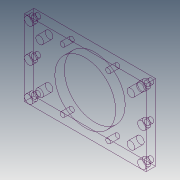
# Autodesk Inventor part: JF-AT-JC0014
Saved by Autodesk Inventor 2015 SP1 (Build 190203100, 203)
## iProperties
Created: 2010-04-29
Part Number: JF-AT-JC0014
Description: Clamper Plate
Document SubType Name: Modeling
Designer: S. Bassin
Density: 2.71 g/cm^3
Material: Aluminum-6061 (Anodized Black)
Mass: 89.7887 g
Surface Area: 133.388 cm^2
Volume: 33.1324 cm^3
Vendor: HHMI: JRC - ID&F
Appearance: Metal-AL-6061 (anodized black)
Revision Number: 0
Autodesk Inventor part; units mm, degrees
ref_plane "YZ Plane" through (0, 0, 0) normal (1, 0, 0) x (0, 1, 0)
ref_plane "XZ Plane" through (0, 0, 0) normal (0, 1, 0) x (-1, 0, 0)
ref_plane "XY Plane" through (0, 0, 0) normal (0, 0, 1) x (1, 0, 0)
sketch "Sketch1" plane through (0, 0, 0) normal (0, 0, 1) x (1, 0, 0)
  line L0 (-21.6696, 43.0812) -> (79.9304, 43.0812)
  line L1 (79.9304, 43.0812) -> (79.9304, -20.4188)
  line L2 (79.9304, -20.4188) -> (-21.6696, -20.4188)
  line L3 (-21.6696, -20.4188) -> (-21.6696, 43.0812)
  point P0 (0, 0)
  dimension "d0" = 101.6
  dimension "d1" = 63.5
  constraints: 8 end point
  measures "d0" distance between parallel lines of L1 L3
  measures "d1" distance between parallel lines of L2 L0
extrude "Extrusion1" add sketch "Sketch1" along normal blind 7.9375
sketch "Sketch3" plane through (0, 0, 7.9375) normal (0, 0, 1) x (1, 0, 0)
  line L0 (-21.6696, 43.0812) -> (79.9304, 43.0812) projected
  line L1 (-21.6696, -20.4188) -> (-21.6696, 43.0812) projected
  point P0 (0, 0)
  point P1 (29.1304, 11.3312)
  dimension "d15" = 31.75
  dimension "d16" = 50.8
  measures "d15" distance from line of L0 point (29.13, 11.331)
  measures "d16" distance from line of L1 point (29.13, 11.331)
hole "Hole2" at (29.1304, 11.3312, 7.9375) direction (0, 0, -1) diameter 50.8 end through all
sketch "Sketch4" plane through (0, 0, 7.9375) normal (0, 0, 1) x (1, 0, 0)
  line L0 (-21.6696, -20.4188) -> (-21.6696, 43.0812) projected
  line L1 (79.9304, -20.4188) -> (-21.6696, -20.4188) projected
  point P0 (0, 0)
  point P1 (10.0804, 36.7312)
  point P2 (10.0804, -14.0688)
  point P3 (48.1804, 36.7312)
  point P4 (48.1804, -14.0688)
  dimension "d24" = 50.8
  dimension "d25" = 6.35
  dimension "d26" = 38.1
  dimension "d27" = 31.75
  dimension "d28" = 31.75
  measures "d24" distance of point (10.08, 36.731) point (10.08, -14.069)
  measures "d25" distance from line of L1 point (10.08, -14.069)
  measures "d26" distance of point (48.18, 36.731) point (10.08, 36.731)
  measures "d27" distance from line of L0 point (10.08, 36.731)
  measures "d28" distance from line of L0 point (10.08, -14.069)
hole "Hole3" at (10.0804, 36.7312, 7.9375) at (10.0804, -14.0688, 7.9375) at (48.1804, 36.7312, 7.9375) at (48.1804, -14.0688, 7.9375) direction (0, 0, -1) diameter 3.9624 end through all thread size "10-32 UNF" class "2B" standard "ANSI Unified Screw Threads"
sketch "Sketch5" plane through (0, 0, 7.9375) normal (0, 0, 1) x (1, 0, 0)
  line L0 (79.9304, 43.0812) -> (79.9304, -20.4188) projected
  line L1 (-21.6696, 43.0812) -> (79.9304, 43.0812) projected
  line L2 (-21.6696, -20.4188) -> (-21.6696, 43.0812) projected
  line L3 (79.9304, -20.4188) -> (-21.6696, -20.4188) projected
  point P0 (0, 0)
  point P1 (-18.1136, 39.5252)
  point P2 (-18.1136, -16.8628)
  point P3 (76.3744, -16.8628)
  point P4 (76.3744, 39.5252)
  point P5 (-18.1136, 11.3312)
  point P6 (76.3744, 11.3312)
  dimension "d36" = 3.556
  dimension "d37" = 3.556
  dimension "d38" = 3.556
  dimension "d39" = 3.556
  dimension "d47" = 3.556
  dimension "d48" = 3.556
  dimension "d49" = 3.556
  dimension "d50" = 3.556
  dimension "d51" = 3.556
  dimension "d52" = 3.556
  dimension "d66" = 94.488
  dimension "d67" = 56.388
  measures "d36" distance from line of L2 point (-18.114, 39.525)
  measures "d37" distance from line of L1 point (-18.114, 39.525)
  measures "d38" distance from line of point (-18.114, -16.863) L3
  measures "d39" distance from line of L0 point (76.374, -16.863)
  measures "d47" distance from line of L2 point (-18.114, -16.863)
  measures "d48" distance from line of L2 point (-18.114, 11.331)
  measures "d49" distance from line of point (76.374, -16.863) L3
  measures "d50" distance from line of point (76.374, 11.331) L0
  measures "d51" distance from line of L0 point (76.374, 39.525)
  measures "d52" horizontal distance of L0.start point (76.374, 39.525)
  measures "d66" horizontal distance of point (76.374, -16.863) point (-18.114, 39.525)
  measures "d67" distance of point (-18.114, -16.863) point (-18.114, 39.525)
hole "Hole4" at (-18.1136, 39.5252, 7.9375) at (-18.1136, -16.8628, 7.9375) at (76.3744, -16.8628, 7.9375) at (76.3744, 39.5252, 7.9375) at (-18.1136, 11.3312, 7.9375) at (76.3744, 11.3312, 7.9375) direction (0, 0, -1) diameter 4.318 end through all counterbore diameter 6.985 counterbore depth 4.1656
sketch "Sketch6" plane through (0, 0, 7.9375) normal (0, 0, 1) x (1, 0, 0)
  line L0 (79.9304, 43.0812) -> (79.9304, -20.4188) projected
  line L1 (-21.6696, 43.0812) -> (79.9304, 43.0812) projected
  line L2 (-21.6696, -20.4188) -> (-21.6696, 43.0812) projected
  line L3 (79.9304, -20.4188) -> (-21.6696, -20.4188) projected
  point P0 (0, 0)
  point P1 (-8.9696, 30.3812)
  point P2 (-8.9696, -7.7188)
  point P3 (67.2304, 30.3812)
  point P4 (67.2304, -7.7188)
  dimension "d53" = 12.7
  dimension "d54" = 12.7
  dimension "d55" = 12.7
  dimension "d56" = 12.7
  dimension "d64" = 12.7
  dimension "d65" = 12.7
  measures "d53" distance from line of L2 point (-8.97, 30.381)
  measures "d54" distance from line of L1 point (-8.97, 30.381)
  measures "d55" distance from line of point (-8.97, -7.719) L3
  measures "d56" distance from line of L0 point (67.23, 30.381)
  measures "d64" distance from line of L2 point (-8.97, -7.719)
  measures "d65" distance from line of point (67.23, -7.719) L0
hole "Hole5" at (-8.9696, 30.3812, 7.9375) at (-8.9696, -7.7188, 7.9375) at (67.2304, 30.3812, 7.9375) at (67.2304, -7.7188, 7.9375) direction (0, 0, -1) diameter 6.4008 end through all thread size "5/16-18 UNC" class "2B" standard "ANSI Unified Screw Threads"
body "Solid1"
